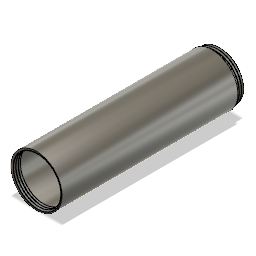
FalconHeavy-BodyTube (Autodesk Fusion 360 design; units mm, degrees)
Autodesk Fusion 360 part; units mm, degrees
sketch "Sketch1" plane through (0, 0, 0) normal (0, 1, 0) x (1, 0, 0)
  line L0 (0, 0) -> (21, 0)
  line L1 (0, 0) -> (20.2, 0)
  line L2 (21, 0) -> (21, 144)
  line L3 (20.2, 0) -> (20.2, 144)
  line L4 (20.2, 144) -> (18.2, 144)
  line L5 (18.2, 144) -> (18.2, 150)
  line L6 (18.2, 150) -> (20.2, 150)
  line L7 (20.2, 150) -> (20.2, 144)
  line L8 (21, 144) -> (20.2, 144)
  line L9 (20.2, 144) -> (20.2, 142)
  spline S0 degree 5 poles (20.2, 142) (20.2, 142.0899) (20.1718, 142.2773) (20.045, 142.5812) (19.7343, 143.0169) (19.2169, 143.5343) (18.7812, 143.845) (18.4773, 143.9718) (18.2899, 144) (18.2, 144) knots 0 0 0 0 0 0 0.2 0.4 0.6 0.8 1 1 1 1 1 1
  line L10 (20.2, 141.8) -> (20.2, 142.2)
  line L11 (18.4, 144) -> (18, 144)
  line L12 (0, 0) -> (0, 150) construction
  line L13 (20.2, 0) -> (20.2, 6)
  line L14 (20.2, 6) -> (0, 6)
  line L15 (20.2, 6) -> (20.2, 7)
  line L16 (20.2, 7) -> (0, 7)
  line L17 (0, 7) -> (0, 6)
  dimension "d1" = 21
  dimension "d2" = 20.2
  dimension "d3" = 144
  dimension "d4" = 144
  dimension "d5" = 2
  dimension "d6" = 6
  dimension "d7" = 2
  dimension "d8" = 2
  dimension "d9" = 150
  dimension "d10" = 6
  dimension "d11" = 1
  constraint coincident L0.start L1.start
  constraint horizontal L0
  constraint parallel L0 L1
  constraint perpendicular L0 L2
  constraint perpendicular L1 L3
  constraint perpendicular L3 L4
  constraint perpendicular L4 L5
  constraint perpendicular L5 L6
  constraint perpendicular L4 L9
  constraint midpoint L9.end L10
  constraint coincident L3 L10.start
  constraint midpoint L4.end L11
  constraint perpendicular L0 L12
  constraint perpendicular L1 L13
  constraint perpendicular L3 L14
  constraint coincident L3 L15.end
  constraint coincident L12 L16.end
  constraint perpendicular L12 L16
  constraint perpendicular L14 L17
  measures "d1" distance of L0.start L0.end
  measures "d2" distance of L0.start L1.end
  measures "d3" distance of L0.end L2.end
  measures "d4" distance of L1.end L3.end
  measures "d5" distance of L3.end L4.end
  measures "d6" distance of L4.end L5.end
  measures "d7" distance of L5.end L6.end
  measures "d8" distance of L3.end L9.end
  measures "d9" distance of L0.start L12.end
  measures "d10" distance of L1.end L13.end
  measures "d11" distance of L13.end L15.end
revolve "Revolve1" add sketch "Sketch1" angle 360 about axis through (0, 0, 0) along (0, 0, -1)
thread "Thread1" "ISO Metric profile 40.0 M40x2 6H" major diameter 40.2565 minor diameter 38.0224 pitch 2 angle 60 modelled right hand crest width 0.25 on face at (19.9384, 3.2403, -2) crest through (19.0112, 0, -7.125)
hole "Hole1" at (0, 0, -6) direction (0, 0, -1) diameter 40.4 depth 20 tip angle 180
thread "Thread2" "ISO Metric profile 40.0 M40x2 6g" major diameter 39.822 minor diameter 37.5289 pitch 2 angle 60 modelled right hand crest width 0.25 on face at (20.1749, -1.0069, -146) crest through (19.911, 0, -150.125)
equation "d2 = 21 mm - Wall_Thickness"
equation "d14 = 42 mm - 2 * Wall_Thickness"
equation "Wall_Thickness = 0.8 mm"
